Autodesk Inventor part; units mm, degrees
(part 2 of 2)
  spline S212 degree 2 poles (3.0927, 10.5084) (3.0556, 10.538) (2.9655, 10.572) (2.9192, 10.572) knots 0 0 0 1 2 2 2
  spline S213 degree 2 poles (2.9192, 10.572) (2.8716, 10.572) (2.8062, 10.5319) (2.8062, 10.4917) knots 0 0 0 1 2 2 2
  spline S214 degree 2 poles (2.8062, 10.4917) (2.8062, 10.4553) (2.8451, 10.4201) (2.8883, 10.409) knots 0 0 0 1 2 2 2
  spline S215 degree 2 poles (2.8883, 10.409) (2.9093, 10.4034) (2.9624, 10.3923) (2.9914, 10.3855) knots 0 0 0 1 2 2 2
  spline S216 degree 2 poles (2.9914, 10.3855) (3.0544, 10.3694) (3.1186, 10.296) (3.1186, 10.2324) knots 0 0 0 1 2 2 2
  spline S217 degree 2 poles (3.1186, 10.2324) (3.1186, 10.1953) (3.0896, 10.1299) (3.0612, 10.1058) knots 0 0 0 1 2 2 2
  spline S218 degree 2 poles (3.0612, 10.1058) (3.0309, 10.0805) (2.9538, 10.0539) (2.8951, 10.0539) knots 0 0 0 1 2 2 2
  line L175 (3.6571, 10.0675) -> (3.5608, 10.0675)
  line L176 (3.5608, 10.0675) -> (3.5608, 10.3935)
  spline S219 degree 2 poles (3.5608, 10.3935) (3.5608, 10.433) (3.5534, 10.501) (3.5422, 10.5214) knots 0 0 0 1 2 2 2
  spline S220 degree 2 poles (3.5422, 10.5214) (3.5305, 10.543) (3.4885, 10.564) (3.4527, 10.564) knots 0 0 0 1 2 2 2
  spline S221 degree 2 poles (3.4527, 10.564) (3.4169, 10.564) (3.3409, 10.5257) (3.3045, 10.4948) knots 0 0 0 1 2 2 2
  line L177 (3.3045, 10.4948) -> (3.3045, 10.0675)
  line L178 (3.3045, 10.0675) -> (3.2082, 10.0675)
  line L179 (3.2082, 10.0675) -> (3.2082, 10.8635)
  line L180 (3.2082, 10.8635) -> (3.3045, 10.8635)
  line L181 (3.3045, 10.8635) -> (3.3045, 10.5757)
  spline S222 degree 2 poles (3.3045, 10.5757) (3.3477, 10.6146) (3.4311, 10.6554) (3.478, 10.6554) knots 0 0 0 1 2 2 2
  spline S223 degree 2 poles (3.478, 10.6554) (3.562, 10.6554) (3.6571, 10.5442) (3.6571, 10.4386) knots 0 0 0 1 2 2 2
  line L182 (3.6571, 10.4386) -> (3.6571, 10.0675)
  line L183 (3.8905, 10.0675) -> (3.7942, 10.0675)
  line L184 (3.7942, 10.0675) -> (3.7942, 10.6393)
  line L185 (3.7942, 10.6393) -> (3.8905, 10.6393)
  line L186 (3.8905, 10.6393) -> (3.8905, 10.0675)
  line L187 (3.8973, 10.7344) -> (3.788, 10.7344)
  line L188 (3.788, 10.7344) -> (3.788, 10.8344)
  line L189 (3.788, 10.8344) -> (3.8973, 10.8344)
  line L190 (3.8973, 10.8344) -> (3.8973, 10.7344)
  line L191 (4.1301, 10.0675) -> (4.0338, 10.0675)
  line L192 (4.0338, 10.0675) -> (4.0338, 10.8635)
  line L193 (4.0338, 10.8635) -> (4.1301, 10.8635)
  line L194 (4.1301, 10.8635) -> (4.1301, 10.0675)
  spline S224 degree 2 poles (4.7507, 10.3688) (4.7507, 10.2256) (4.6142, 10.0564) (4.5099, 10.0564) knots 0 0 0 1 2 2 2
  spline S225 degree 2 poles (4.5099, 10.0564) (4.4673, 10.0564) (4.4018, 10.0761) (4.3678, 10.0965) knots 0 0 0 1 2 2 2
  line L195 (4.3678, 10.0965) -> (4.3678, 9.8569)
  line L196 (4.3678, 9.8569) -> (4.2715, 9.8569)
  line L197 (4.2715, 9.8569) -> (4.2715, 10.6393)
  line L198 (4.2715, 10.6393) -> (4.3678, 10.6393)
  line L199 (4.3678, 10.6393) -> (4.3678, 10.5794)
  spline S226 degree 2 poles (4.3678, 10.5794) (4.4037, 10.6121) (4.4913, 10.6554) (4.5426, 10.6554) knots 0 0 0 1 2 2 2
  spline S227 degree 2 poles (4.5426, 10.6554) (4.6408, 10.6554) (4.7507, 10.4997) (4.7507, 10.3688) knots 0 0 0 1 2 2 2
  spline S228 degree 2 poles (4.6513, 10.3577) (4.6513, 10.4559) (4.5889, 10.564) (4.5191, 10.564) knots 0 0 0 1 2 2 2
  spline S229 degree 2 poles (4.5191, 10.564) (4.4784, 10.564) (4.4018, 10.5275) (4.3678, 10.4991) knots 0 0 0 1 2 2 2
  line L200 (4.3678, 10.4991) -> (4.3678, 10.1743)
  spline S230 degree 2 poles (4.3678, 10.1743) (4.4055, 10.1564) (4.4592, 10.1428) (4.4938, 10.1428) knots 0 0 0 1 2 2 2
  spline S231 degree 2 poles (4.4938, 10.1428) (4.5685, 10.1428) (4.6513, 10.2527) (4.6513, 10.3577) knots 0 0 0 1 2 2 2
  spline S232 degree 2 poles (5.1694, 10.128) (5.1576, 10.1194) (5.1181, 10.0885) (5.0996, 10.0792) knots 0 0 0 1 2 2 2
  spline S233 degree 2 poles (5.0996, 10.0792) (5.0743, 10.0656) (5.0267, 10.0514) (4.9835, 10.0514) knots 0 0 0 1 2 2 2
  spline S234 degree 2 poles (4.9835, 10.0514) (4.9483, 10.0514) (4.8847, 10.078) (4.8606, 10.1021) knots 0 0 0 1 2 2 2
  spline S235 degree 2 poles (4.8606, 10.1021) (4.8378, 10.1255) (4.81, 10.1947) (4.81, 10.233) knots 0 0 0 1 2 2 2
  spline S236 degree 2 poles (4.81, 10.233) (4.81, 10.2923) (4.86, 10.3762) (4.9143, 10.4003) knots 0 0 0 1 2 2 2
  spline S237 degree 2 poles (4.9143, 10.4003) (4.9625, 10.4226) (5.0934, 10.4392) (5.1694, 10.4435) knots 0 0 0 1 2 2 2
  line L201 (5.1694, 10.4435) -> (5.1694, 10.4621)
  spline S238 degree 2 poles (5.1694, 10.4621) (5.1694, 10.4954) (5.149, 10.5368) (5.1305, 10.5485) knots 0 0 0 1 2 2 2
  spline S239 degree 2 poles (5.1305, 10.5485) (5.1119, 10.5603) (5.0588, 10.5677) (5.0304, 10.5677) knots 0 0 0 1 2 2 2
  spline S240 degree 2 poles (5.0304, 10.5677) (4.9971, 10.5677) (4.9069, 10.5479) (4.8618, 10.5288) knots 0 0 0 1 2 2 2
  line L202 (4.8618, 10.5288) -> (4.8563, 10.5288)
  line L203 (4.8563, 10.5288) -> (4.8563, 10.6269)
  spline S241 degree 2 poles (4.8563, 10.6269) (4.8828, 10.6344) (4.9823, 10.6529) (5.031, 10.6529) knots 0 0 0 1 2 2 2
  spline S242 degree 2 poles (5.031, 10.6529) (5.0903, 10.6529) (5.1712, 10.6344) (5.2033, 10.6103) knots 0 0 0 1 2 2 2
  spline S243 degree 2 poles (5.2033, 10.6103) (5.2348, 10.5868) (5.2657, 10.5121) (5.2657, 10.4584) knots 0 0 0 1 2 2 2
  line L204 (5.2657, 10.4584) -> (5.2657, 10.0675)
  line L205 (5.2657, 10.0675) -> (5.1694, 10.0675)
  line L206 (5.1694, 10.0675) -> (5.1694, 10.128)
  line L207 (5.1694, 10.2083) -> (5.1694, 10.367)
  spline S244 degree 2 poles (5.1694, 10.367) (5.1348, 10.3639) (5.0304, 10.3534) (4.9977, 10.3435) knots 0 0 0 1 2 2 2
  spline S245 degree 2 poles (4.9977, 10.3435) (4.9594, 10.3318) (4.9094, 10.283) (4.9094, 10.2398) knots 0 0 0 1 2 2 2
  spline S246 degree 2 poles (4.9094, 10.2398) (4.9094, 10.1904) (4.965, 10.1404) (5.0181, 10.1404) knots 0 0 0 1 2 2 2
  spline S247 degree 2 poles (5.0181, 10.1404) (5.0632, 10.1404) (5.1373, 10.1793) (5.1694, 10.2083) knots 0 0 0 1 2 2 2
  spline S248 degree 2 poles (5.5738, 10.0564) (5.4954, 10.0564) (5.4071, 10.1459) (5.4071, 10.2429) knots 0 0 0 1 2 2 2
  line L208 (5.4071, 10.2429) -> (5.4071, 10.5596)
  line L209 (5.4071, 10.5596) -> (5.3423, 10.5596)
  line L210 (5.3423, 10.5596) -> (5.3423, 10.6393)
  line L211 (5.3423, 10.6393) -> (5.4071, 10.6393)
  line L212 (5.4071, 10.6393) -> (5.4071, 10.8036)
  line L213 (5.4071, 10.8036) -> (5.5034, 10.8036)
  line L214 (5.5034, 10.8036) -> (5.5034, 10.6393)
  line L215 (5.5034, 10.6393) -> (5.6807, 10.6393)
  line L216 (5.6807, 10.6393) -> (5.6807, 10.5596)
  line L217 (5.6807, 10.5596) -> (5.5034, 10.5596)
  line L218 (5.5034, 10.5596) -> (5.5034, 10.2873)
  spline S249 degree 2 poles (5.5034, 10.2873) (5.5034, 10.2441) (5.5065, 10.1965) (5.517, 10.1762) knots 0 0 0 1 2 2 2
  spline S250 degree 2 poles (5.517, 10.1762) (5.5257, 10.1583) (5.5646, 10.1404) (5.5979, 10.1404) knots 0 0 0 1 2 2 2
  spline S251 degree 2 poles (5.5979, 10.1404) (5.6214, 10.1404) (5.6652, 10.1546) (5.6751, 10.1589) knots 0 0 0 1 2 2 2
  line L219 (5.6751, 10.1589) -> (5.6807, 10.1589)
  line L220 (5.6807, 10.1589) -> (5.6807, 10.0724)
  spline S252 degree 2 poles (5.6807, 10.0724) (5.6535, 10.065) (5.5979, 10.0564) (5.5738, 10.0564) knots 0 0 0 1 2 2 2
  spline S253 degree 2 poles (5.9999, 10.0545) (5.8628, 10.0545) (5.7122, 10.2083) (5.7122, 10.3503) knots 0 0 0 1 2 2 2
  spline S254 degree 2 poles (5.7122, 10.3503) (5.7122, 10.4899) (5.8585, 10.6554) (5.9764, 10.6554) knots 0 0 0 1 2 2 2
  spline S255 degree 2 poles (5.9764, 10.6554) (6.0295, 10.6554) (6.1117, 10.6245) (6.1419, 10.5917) knots 0 0 0 1 2 2 2
  spline S256 degree 2 poles (6.1419, 10.5917) (6.1728, 10.559) (6.2055, 10.4645) (6.2055, 10.396) knots 0 0 0 1 2 2 2
  line L221 (6.2055, 10.396) -> (6.2055, 10.3435)
  line L222 (6.2055, 10.3435) -> (5.8097, 10.3435)
  spline S257 degree 2 poles (5.8097, 10.3435) (5.8097, 10.2441) (5.9098, 10.1385) (5.9987, 10.1385) knots 0 0 0 1 2 2 2
  spline S258 degree 2 poles (5.9987, 10.1385) (6.0302, 10.1385) (6.0913, 10.1527) (6.116, 10.1638) knots 0 0 0 1 2 2 2
  spline S259 degree 2 poles (6.116, 10.1638) (6.1419, 10.1762) (6.1777, 10.1978) (6.1895, 10.2077) knots 0 0 0 1 2 2 2
  line L223 (6.1895, 10.2077) -> (6.195, 10.2077)
  line L224 (6.195, 10.2077) -> (6.195, 10.1027)
  spline S260 degree 2 poles (6.195, 10.1027) (6.1784, 10.0959) (6.1277, 10.0761) (6.108, 10.0706) knots 0 0 0 1 2 2 2
  spline S261 degree 2 poles (6.108, 10.0706) (6.0802, 10.0625) (6.0345, 10.0545) (5.9999, 10.0545) knots 0 0 0 1 2 2 2
  spline S262 degree 2 poles (6.1117, 10.417) (6.1104, 10.4559) (6.0944, 10.5127) (6.0789, 10.5319) knots 0 0 0 1 2 2 2
  spline S263 degree 2 poles (6.0789, 10.5319) (6.0623, 10.5535) (6.0098, 10.5763) (5.9709, 10.5763) knots 0 0 0 1 2 2 2
  spline S264 degree 2 poles (5.9709, 10.5763) (5.9326, 10.5763) (5.8789, 10.5535) (5.8566, 10.5312) knots 0 0 0 1 2 2 2
  spline S265 degree 2 poles (5.8566, 10.5312) (5.835, 10.5084) (5.8128, 10.4534) (5.8097, 10.417) knots 0 0 0 1 2 2 2
  line L225 (5.8097, 10.417) -> (6.1117, 10.417)
  line L226 (6.4013, 10.0675) -> (6.305, 10.0675)
  line L227 (6.305, 10.0675) -> (6.305, 10.8635)
  line L228 (6.305, 10.8635) -> (6.4013, 10.8635)
  line L229 (6.4013, 10.8635) -> (6.4013, 10.0675)
  line L230 (6.6921, 10.0675) -> (6.5699, 10.0675)
  line L231 (6.5699, 10.0675) -> (6.5699, 10.2132)
  line L232 (6.5699, 10.2132) -> (6.6921, 10.2132)
  line L233 (6.6921, 10.2132) -> (6.6921, 10.0675)
  spline S266 degree 2 poles (7.0873, 10.0545) (7.0281, 10.0545) (6.9299, 10.091) (6.8947, 10.128) knots 0 0 0 1 2 2 2
  spline S267 degree 2 poles (6.8947, 10.128) (6.8595, 10.1644) (6.8206, 10.2768) (6.8206, 10.3522) knots 0 0 0 1 2 2 2
  spline S268 degree 2 poles (6.8206, 10.3522) (6.8206, 10.4275) (6.8607, 10.5374) (6.8947, 10.5745) knots 0 0 0 1 2 2 2
  spline S269 degree 2 poles (6.8947, 10.5745) (6.9286, 10.6121) (7.0293, 10.6523) (7.0873, 10.6523) knots 0 0 0 1 2 2 2
  spline S270 degree 2 poles (7.0873, 10.6523) (7.1343, 10.6523) (7.2219, 10.6257) (7.2559, 10.6084) knots 0 0 0 1 2 2 2
  line L234 (7.2559, 10.6084) -> (7.2559, 10.5004)
  line L235 (7.2559, 10.5004) -> (7.2504, 10.5004)
  spline S271 degree 2 poles (7.2504, 10.5004) (7.2399, 10.509) (7.2077, 10.5312) (7.1849, 10.543) knots 0 0 0 1 2 2 2
  spline S272 degree 2 poles (7.1849, 10.543) (7.1645, 10.5528) (7.1102, 10.5683) (7.0855, 10.5683) knots 0 0 0 1 2 2 2
  spline S273 degree 2 poles (7.0855, 10.5683) (7.0108, 10.5683) (6.92, 10.4553) (6.92, 10.3522) knots 0 0 0 1 2 2 2
  spline S274 degree 2 poles (6.92, 10.3522) (6.92, 10.2515) (7.0077, 10.1385) (7.0855, 10.1385) knots 0 0 0 1 2 2 2
  spline S275 degree 2 poles (7.0855, 10.1385) (7.1324, 10.1385) (7.2176, 10.1774) (7.2504, 10.2077) knots 0 0 0 1 2 2 2
  line L236 (7.2504, 10.2077) -> (7.2559, 10.2077)
  line L237 (7.2559, 10.2077) -> (7.2559, 10.0996)
  spline S276 degree 2 poles (7.2559, 10.0996) (7.2417, 10.0928) (7.1985, 10.0737) (7.1812, 10.0693) knots 0 0 0 1 2 2 2
  spline S277 degree 2 poles (7.1812, 10.0693) (7.1565, 10.0619) (7.1176, 10.0545) (7.0873, 10.0545) knots 0 0 0 1 2 2 2
  spline S278 degree 2 poles (7.8135, 10.3534) (7.8135, 10.2089) (7.6746, 10.0514) (7.5585, 10.0514) knots 0 0 0 1 2 2 2
  spline S279 degree 2 poles (7.5585, 10.0514) (7.4393, 10.0514) (7.3028, 10.2138) (7.3028, 10.3534) knots 0 0 0 1 2 2 2
  spline S280 degree 2 poles (7.3028, 10.3534) (7.3028, 10.4967) (7.4436, 10.6554) (7.5585, 10.6554) knots 0 0 0 1 2 2 2
  spline S281 degree 2 poles (7.5585, 10.6554) (7.6746, 10.6554) (7.8135, 10.4973) (7.8135, 10.3534) knots 0 0 0 1 2 2 2
  spline S282 degree 2 poles (7.7141, 10.3534) (7.7141, 10.4645) (7.6332, 10.5726) (7.5585, 10.5726) knots 0 0 0 1 2 2 2
  spline S283 degree 2 poles (7.5585, 10.5726) (7.4838, 10.5726) (7.4023, 10.4645) (7.4023, 10.3534) knots 0 0 0 1 2 2 2
  spline S284 degree 2 poles (7.4023, 10.3534) (7.4023, 10.2453) (7.4838, 10.1342) (7.5585, 10.1342) knots 0 0 0 1 2 2 2
  spline S285 degree 2 poles (7.5585, 10.1342) (7.6326, 10.1342) (7.7141, 10.2435) (7.7141, 10.3534) knots 0 0 0 1 2 2 2
  line L238 (8.5607, 10.0675) -> (8.5607, 10.3985)
  spline S286 degree 2 poles (8.5607, 10.3985) (8.5607, 10.438) (8.5545, 10.5053) (8.5446, 10.5238) knots 0 0 0 1 2 2 2
  spline S287 degree 2 poles (8.5446, 10.5238) (8.5348, 10.5442) (8.4971, 10.564) (8.4644, 10.564) knots 0 0 0 1 2 2 2
  spline S288 degree 2 poles (8.4644, 10.564) (8.4347, 10.564) (8.3668, 10.5275) (8.331, 10.4929) knots 0 0 0 1 2 2 2
  spline S289 degree 2 poles (8.331, 10.4929) (8.3316, 10.4843) (8.3328, 10.4602) (8.3328, 10.4442) knots 0 0 0 1 2 2 2
  line L239 (8.3328, 10.4442) -> (8.3328, 10.0675)
  line L240 (8.3328, 10.0675) -> (8.2365, 10.0675)
  line L241 (8.2365, 10.0675) -> (8.2365, 10.3985)
  spline S290 degree 2 poles (8.2365, 10.3985) (8.2365, 10.438) (8.2303, 10.5053) (8.2205, 10.5238) knots 0 0 0 1 2 2 2
  spline S291 degree 2 poles (8.2205, 10.5238) (8.2106, 10.5442) (8.1729, 10.564) (8.1402, 10.564) knots 0 0 0 1 2 2 2
  spline S292 degree 2 poles (8.1402, 10.564) (8.1093, 10.564) (8.0408, 10.5251) (8.0086, 10.4948) knots 0 0 0 1 2 2 2
  line L242 (8.0086, 10.4948) -> (8.0086, 10.0675)
  line L243 (8.0086, 10.0675) -> (7.9123, 10.0675)
  line L244 (7.9123, 10.0675) -> (7.9123, 10.6393)
  line L245 (7.9123, 10.6393) -> (8.0086, 10.6393)
  line L246 (8.0086, 10.6393) -> (8.0086, 10.5763)
  spline S293 degree 2 poles (8.0086, 10.5763) (8.0463, 10.614) (8.1204, 10.6554) (8.1649, 10.6554) knots 0 0 0 1 2 2 2
  spline S294 degree 2 poles (8.1649, 10.6554) (8.2155, 10.6554) (8.2939, 10.609) (8.3143, 10.5566) knots 0 0 0 1 2 2 2
  spline S295 degree 2 poles (8.3143, 10.5566) (8.3582, 10.6053) (8.4409, 10.6554) (8.4891, 10.6554) knots 0 0 0 1 2 2 2
  spline S296 degree 2 poles (8.4891, 10.6554) (8.5261, 10.6554) (8.5866, 10.6325) (8.6089, 10.6066) knots 0 0 0 1 2 2 2
  spline S297 degree 2 poles (8.6089, 10.6066) (8.6317, 10.5806) (8.657, 10.5028) (8.657, 10.4442) knots 0 0 0 1 2 2 2
  line L247 (8.657, 10.4442) -> (8.657, 10.0675)
  line L248 (8.657, 10.0675) -> (8.5607, 10.0675)
  point P0 (-14.605, -4.445)
  constraints: 2 other
emboss "Emboss2" sketch "Sketch24" operation cut depth 0.762 direction (-1, 0, 0)
body "Solid1"
